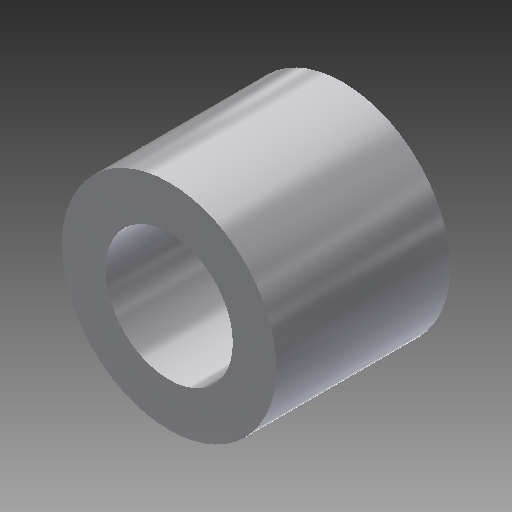
# Autodesk Inventor part: ナイロンスペーサー(中空）外径3.7内径2.2長3_CN-2003
Saved by Autodesk Inventor 2017 (Build 210142000, 142)
## iProperties
Created: 2013-09-26
Part Number: ナイロンスペーサー(中空）外径3.7内径2.2長3_CN-2003
Document SubType Name: Modeling
Designer: NN
Density: 1.06 g/cm^3
Material: ABS Plastic
Mass: 0.0221035 g
Surface Area: 0.695077 cm^2
Volume: 0.0208523 cm^3
Appearance: 滑らか - 白
Author: NN
Autodesk Inventor part; units mm, degrees
ref_plane "YZ Plane" through (0, 0, 0) normal (1, 0, 0) x (0, 1, 0)
ref_plane "XZ Plane" through (0, 0, 0) normal (0, 1, 0) x (-1, 0, 0)
ref_plane "XY Plane" through (0, 0, 0) normal (0, 0, 1) x (1, 0, 0)
sketch "スケッチ1" plane through (0, 0, 0) normal (0, 0, 1) x (1, 0, 0)
  circle A0 centre (0, 0) radius 1.1
  circle A1 centre (0, 0) radius 1.85
  dimension "d0" = 2.2
  dimension "d1" = 3.7
  constraints: 2 centre point, 2 coincident
  measures "d0" diameter of A0
  measures "d1" diameter of A1
extrude "押し出し1" add sketch "スケッチ1" along normal blind 3
